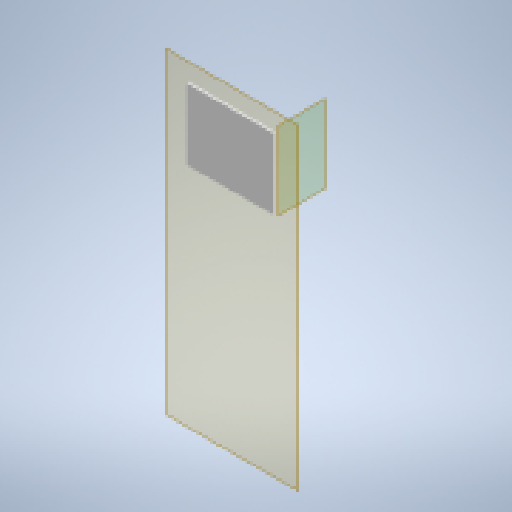
# Autodesk Inventor part: задняя часть спины
Saved by Autodesk Inventor 2024.2 (Build 282272000, 272)
## iProperties
Created: 2025-10-07
Part Number: задняя часть спины
Material: Типовые
Document SubType Name: Modeling
Designer: katya_notebook
Density: 1 g/cm^3
Appearance: По умолчанию
Author: katya_notebook
Autodesk Inventor part; units mm, degrees
ref_plane "YZ Plane" through (0, 0, 0) normal (1, 0, 0) x (0, 1, 0)
ref_plane "XZ Plane" through (0, 0, 0) normal (0, 1, 0) x (-1, 0, 0)
ref_plane "РабПлоскость1" through (0, 0, 0) normal (0, 0, 1) x (1, 0, 0)
ref_plane "РабПлоскость2" through (-9.7, 217.1229, -41) normal (-1, 0, 0) x (0, -1, 0)
ref_plane "РабПлоскость3" through (-83.5, 156.7629, -36.5) normal (1, 0, 0) x (0, 1, 0)
sketch "Эскиз2" plane through (-9.7, 217.1229, -41) normal (-1, 0, 0) x (0, -1, 0)
  line L0 (0, 0) -> (0, 41) projected
  line L1 (61.68, 0) -> (61.68, 39) projected
  line L2 (60.36, 0) -> (60.36, 41) projected
  line L3 (0, 41) -> (0, 43)
  line L4 (0, 43) -> (60.36, 43)
  line L5 (60.36, 41) -> (60.36, 43)
  line L6 (0, 41) -> (60.36, 41)
  point P0 (217.1229, 41)
  dimension "d0" = 2
  constraints: 8 end point, 2 perpendicular, 2 point on line, 1 collinear
  measures "d0" distance of L0.end L3.end
extrude "Выдавливание1" add sketch "Эскиз2" along normal up to surface (73.8 mm away)
